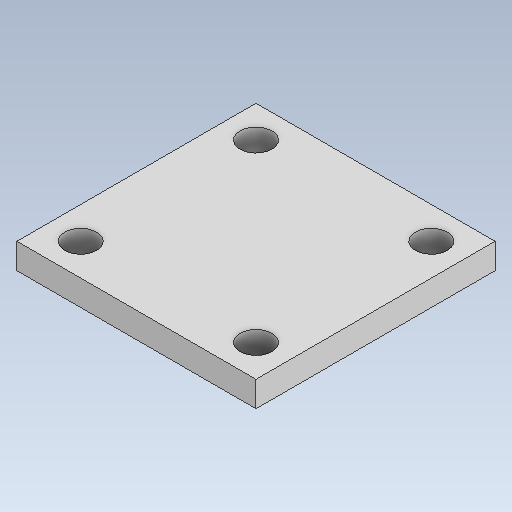
# Autodesk Inventor part: encoder_pcb
Saved by Autodesk Inventor 2020 (Build 240168000, 168)
## iProperties
Created: 2019-05-15
Part Number: encoder_pcb
Material: Generic
Document SubType Name: Modeling
Designer: psrob
Density: 1 g/cm^3
Appearance: Default
Author: psrob
Autodesk Inventor part; units mm, degrees
ref_plane "YZ Plane" through (0, 0, 0) normal (1, 0, 0) x (0, 1, 0)
ref_plane "XZ Plane" through (0, 0, 0) normal (0, 1, 0) x (-1, 0, 0)
ref_plane "XY Plane" through (0, 0, 0) normal (0, 0, 1) x (1, 0, 0)
sketch "Sketch1" plane through (0, 0, 0) normal (0, 1, 0) x (-1, 0, 0)
  line L0 (5.5, 5.5) -> (5.5, -5.5)
  line L1 (5.5, -5.5) -> (-5.5, -5.5)
  line L2 (-5.5, -5.5) -> (-5.5, 5.5)
  line L3 (-5.5, 5.5) -> (5.5, 5.5)
  line L4 (5.5, 5.5) -> (-5.5, -5.5) construction
  line L5 (5.5, -5.5) -> (-5.5, 5.5) construction
  circle A0 centre (5.5, 5.5) radius 1
  circle A1 centre (5.5, -5.5) radius 1
  circle A2 centre (-5.5, 5.5) radius 1
  circle A3 centre (-5.5, -5.5) radius 1
  line L6 (7.5, 7.5) -> (7.5, -7.5)
  line L7 (7.5, -7.5) -> (-7.5, -7.5)
  line L8 (-7.5, -7.5) -> (-7.5, 7.5)
  line L9 (-7.5, 7.5) -> (7.5, 7.5)
  line L10 (7.5, 7.5) -> (-7.5, -7.5) construction
  line L11 (7.5, -7.5) -> (-7.5, 7.5) construction
  point P0 (0, 0)
  dimension "d0" = 11
  dimension "d1" = 11
  dimension "d2" = 2
  dimension "d3" = 2
  dimension "d4" = 2
  dimension "d5" = 2
  dimension "d6" = 15
  dimension "d7" = 15
  constraints: 24 end point, 4 centre point, 4 coincident, 4 midpoint, 4 parallel, 2 perpendicular, 2 vertical
  measures "d0" distance of L0.start L0.end
  measures "d1" distance of L0.end L1.end
  measures "d2" diameter of A0
  measures "d3" diameter of A1
  measures "d4" diameter of A2
  measures "d5" diameter of A3
  measures "d6" distance of L6.start L6.end
  measures "d7" distance of L8.end L6.start
extrude "Extrusion1" add sketch "Sketch1" along normal blind 1.6 contours L0 A1 L1 A3 L2 A2 L3 A0 | L6 L7 L8 L9
body "Solid1"
